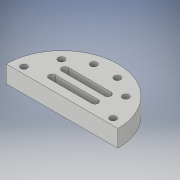
# Autodesk Inventor part: PVC_WireAnchor
Saved by Autodesk Inventor 2019 (Build 230136000, 136)
## iProperties
Created: 2018-09-02
Part Number: PVC_WireAnchor
Material: Generic
Document SubType Name: Modeling
Designer: Crater-Windows
Density: 1 g/cm^3
Appearance: Default
Author: Crater-Windows
Autodesk Inventor part; units mm, degrees
ref_plane "YZ Plane" through (0, 0, 0) normal (1, 0, 0) x (0, 1, 0)
ref_plane "XZ Plane" through (0, 0, 0) normal (0, 1, 0) x (-1, 0, 0)
ref_plane "XY Plane" through (0, 0, 0) normal (0, 0, 1) x (1, 0, 0)
sketch "Sketch1" plane through (0, 0, 0) normal (0, 1, 0) x (-1, 0, 0)
  line L0 (0, 0) -> (-51.9938, 0)
  arc A0 (-51.9938, 0) -> (0, 0) centre (-25.9969, 0) ccw
  dimension "d0" = 51.9938
  dimension "d1" = 25.9969
  constraints: 2 end point, 2 point on circle, 1 centre point, 1 horizontal
  measures "d0" distance of L0.start L0.end
  measures "d1" radius of A0
extrude "Extrusion1" add sketch "Sketch1" along normal blind 8
sketch "Sketch2" plane through (0, 8, 0) normal (0, 1, 0) x (1, 0, 0)
  line L0 (5.2154, 3) -> (46.7784, 3)
  line L1 (0, 0) -> (51.9938, 0) projected
  arc A0 (46.7784, 3) -> (5.2154, 3) centre (25.9969, 0) ccw
  arc A1 (51.9938, 0) -> (0, 0) centre (25.9969, 0) ccw projected
  arc A2 (37.6159, 3) -> (14.3779, 3) centre (25.9969, 0) ccw
  line L2 (7.8131, 10.4985) -> (15.6046, 6) construction
  line L3 (16.8902, 18.9192) -> (14.7121, 4.0808) construction
  line L4 (25.9969, 20.9969) -> (25.9969, 12) construction
  line L5 (34.1779, 19.3375) -> (37.4243, 3.6625) construction
  line L6 (36.3892, 6) -> (44.1807, 10.4984) construction
  circle A3 centre (5.2154, 3) radius 1.5
  circle A4 centre (10.9969, 14.6925) radius 1.5
  circle A5 centre (20.4969, 20.2638) radius 1.5
  circle A6 centre (31.4969, 20.2638) radius 1.5
  circle A7 centre (40.9969, 14.6925) radius 1.5
  circle A8 centre (46.7784, 3) radius 1.5
  line L7 (15.8011, 11.5) -> (35.8011, 11.5) construction
  line L8 (15.8011, 10) -> (35.8011, 10)
  line L9 (35.8011, 13) -> (15.8011, 13)
  arc A9 (15.8011, 13) -> (15.8011, 10) centre (15.8011, 11.5) ccw
  arc A10 (35.8011, 10) -> (35.8011, 13) centre (35.8011, 11.5) ccw
  line L10 (15.8011, 5.5) -> (35.8011, 5.5) construction
  line L11 (15.8011, 4) -> (35.8011, 4)
  line L12 (35.8011, 7) -> (15.8011, 7)
  arc A11 (15.8011, 7) -> (15.8011, 4) centre (15.8011, 5.5) ccw
  arc A12 (35.8011, 4) -> (35.8011, 7) centre (35.8011, 5.5) ccw
  point P0 (25.9969, 0)
  point P1 (11.7088, 8.2492)
  point P2 (25.9969, 16.4985)
  point P3 (40.285, 8.2492)
  point P4 (25.8011, 11.5)
  point P5 (25.8011, 5.5)
  dimension "d4" = 3
  dimension "d5" = 5
  dimension "d6" = 12
  dimension "d15" = 3
  dimension "d16" = 3
  dimension "d17" = 3
  dimension "d18" = 3
  dimension "d19" = 3
  dimension "d21" = 3
  dimension "d22" = 11
  dimension "d23" = 30
  dimension "d24" = 3
  dimension "d25" = 3
  dimension "d26" = 3
  dimension "d27" = 4
  dimension "d28" = 20
  constraints: 38 end point, 15 point on circle, 11 centre point, 8 midpoint, 8 tangent, 4 coincident, 4 parallel, 2 horizontal, 2 horizontal alignment, 2 point on line, 1 vertical alignment, 14 other
  measures "d4" distance between parallel lines of L0 L1
  measures "d6" radius of A2
  measures "d15" diameter of A3
  measures "d16" diameter of A4
  measures "d17" diameter of A5
  measures "d18" diameter of A6
  measures "d19" diameter of A7
  measures "d21" diameter of A8
  measures "d22" distance of A6.centre A5.centre
  measures "d23" distance of A7.centre A4.centre
  measures "d24" diameter of A10
  measures "d25" diameter of A12
  measures "d26" distance between parallel lines of L12 L8
  measures "d27" distance between parallel lines of L1 L11
  measures "d28" distance of L7.end L7.start
extrude "Extrusion2" cut sketch "Sketch2" against normal blind 15 contours A0 A3 L0 | L0 A3 A0 | A4 A0 | A0 A4 | A11 L12 A2 | A2 L12 A12 L11 A11 | A8 A0 L0 | L0 A0 A8 | A2 L12 A12 | A5 A0 | A0 A5 | L8 A9 L9 A10 A2 | A2 L8 | A7 A0 | A0 A7 | A6 A0 | A0 A6
equation "\"d1\" = 0.5 * d0"
body "Solid1"
